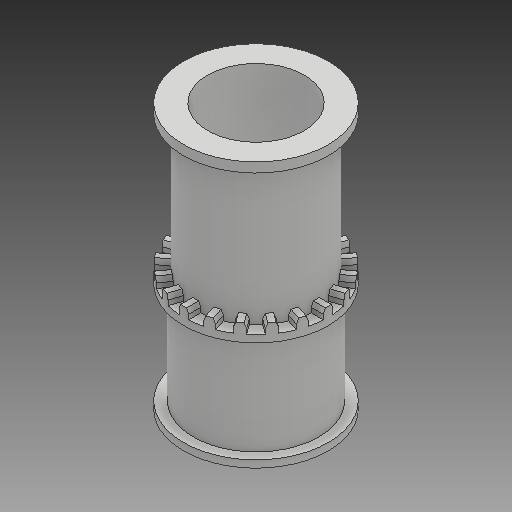
# Autodesk Inventor part: Rigid holder
Saved by Autodesk Inventor 2018 (Build 220112000, 112)
## iProperties
Created: 2016-02-19
Part Number: Rigid holder
Material: Generic
Document SubType Name: Modeling
Designer: Tore Den Store
Density: 1 g/cm^3
Appearance: Default
Author: Tore Den Store
Autodesk Inventor part; units mm, degrees
ref_plane "YZ Plane" through (0, 0, 0) normal (1, 0, 0) x (0, 1, 0)
sketch "Sketch1" plane through (0, 0, 0) normal (0, 0, 1) x (1, 0, 0)
  circle A0 centre (0, 0) radius 130
  dimension "d0" = 260
  constraints: 1 centre point, 1 coincident
  measures "d0" diameter of A0
extrude "Extrusion1" add sketch "Sketch1" along normal blind 210
sketch "Sketch2" plane through (0, 0, 210) normal (0, 0, 1) x (1, 0, 0)
  circle A0 centre (0, 0) radius 150
  dimension "d3" = 300
  constraints: 1 centre point, 1 coincident
  measures "d3" diameter of A0
extrude "Extrusion2" add sketch "Sketch2" along normal blind 15
ref_plane "Work Plane3" through (0, 0, 105) normal (0, 0, -1) x (-1, 0, 0)
mirror "Mirror2" about plane through (0, 0, 105) normal (0, 0, -1) of "Extrusion2"
hole "Hole2" at (0, 0, 225) direction (0, 0, -1) diameter 200 end through all
sketch "Sketch7" plane through (0, 0, 225) normal (0, 0, 1) x (1, 0, 0)
  circle A0 centre (0, 0) radius 100 projected
  circle A1 centre (0, 0) radius 100 projected
  circle A2 centre (0, 0) radius 150 projected
  line L0 (0, 0) -> (-9.8074, -124.6147) construction
  circle A3 centre (0, 0) radius 150 projected
  line L1 (0, 0) -> (154.8223, 0) construction
  line L2 (0, 0) -> (9.8074, -124.6147) construction
  line L3 (-9.8074, -124.6147) -> (-9.8074, -149.679)
  line L4 (9.8074, -124.6147) -> (9.8074, -149.679)
  circle A4 centre (0, 0) radius 125
  dimension "d40" = 94.5
  dimension "d41" = 9
  dimension "d73" = 250
  constraints: 10 end point, 6 point on circle, 2 vertical, 1 centre point, 1 coincident, 1 horizontal
  measures "d40" angle of L0 L1
  measures "d41" angle of L2 L0
  measures "d73" diameter of A4
extrude "Extrusion7" add sketch "Sketch7" along normal blind 20 contours L3 A4 L4 A2 picked at (-7.629, -133.0836)
ref_plane "Work Plane4" through (-9.8074, -149.679, 225) normal (0, 1, 0) x (0, 0, 1)
sketch "Sketch8" plane through (-9.8074, -149.679, 225) normal (0, 1, 0) x (0, 0, 1)
  line L0 (20, 0) -> (10, 0)
  line L1 (0, 0) -> (20, 0) projected
  line L2 (20, 0) -> (20, 3.6397)
  line L3 (10, 0) -> (20, 3.6397)
  line L4 (0, 19.6148) -> (20, 19.6148) projected
  line L5 (20, 19.6148) -> (10, 19.6148)
  line L6 (10, 19.6148) -> (20, 15.9751)
  line L7 (20, 15.9751) -> (20, 19.6148)
  line L8 (20, 0) -> (20, 19.6148) projected
  line L9 (0, -140.1926) -> (0, 159.8074) projected
  point P0 (-225, 9.8074)
  point P1 (0, 20.3994)
  dimension "d49" = 10
  dimension "d50" = 20
  dimension "d52" = 10
  dimension "d53" = 20
  constraints: 12 end point, 2 point on line, 1 midpoint, 2 other
  measures "d49" distance of L0.start L0.end
  measures "d50" angle of L3 L0
  measures "d52" distance of L5.start L5.end
  measures "d53" angle to the sketch x axis of L6
extrude "Extrusion8" cut sketch "Sketch8" along normal through all both and the other way through all contours L0 L3 L2 | L6 L4 L7
pattern_circular "Circular Pattern2" count 20 over 360 about axis through (0, 0, -262.4423) along (0, 0, 1) of "Extrusion7", "Extrusion8"
sketch "Sketch10" plane through (0, 0, 225) normal (0, 0, 1) x (1, 0, 0)
  circle A0 centre (0, 0) radius 100 projected
  circle A1 centre (0, 0) radius 125
  dimension "d64" = 25
  constraints: 1 centre point
  measures "d64" radial gap between concentric circles of A0 A1
extrude "Extrusion10" add sketch "Sketch10" along normal blind 290
sketch "Sketch12" plane through (0, 0, 515) normal (0, 0, 1) x (1, 0, 0)
  circle A0 centre (0, 0) radius 150
  circle A1 centre (0, 0) radius 100 projected
  dimension "d70" = 300
  constraints: 1 centre point, 1 coincident
  measures "d70" diameter of A0
extrude "Extrusion12" add sketch "Sketch12" along normal blind 20
equation "\"d52\" = d49"
equation "\"d53\" = d50"
body "Solid1"
